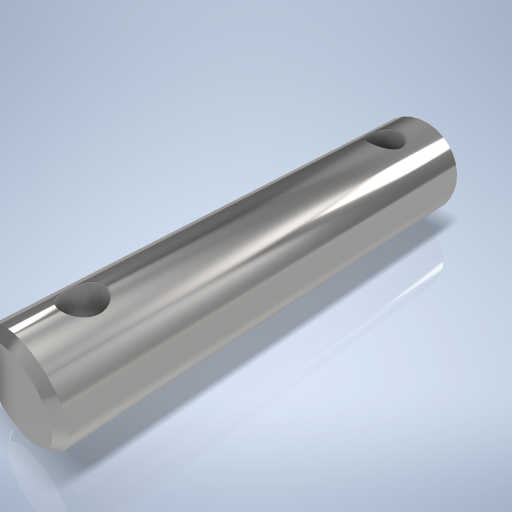
# Autodesk Inventor part: BMS_bolts_left
Saved by Autodesk Inventor 2024.2 (Build 282272000, 272)
## iProperties
Created: 2024-05-14
Part Number: BMS_bolts_left
Material: Edelstahl
Document SubType Name: Modeling
Designer: Fabri
Density: 8 g/cm^3
Appearance: Kordiert 45
Author: Fabri
Autodesk Inventor part; units mm, degrees
ref_plane "YZ Plane" through (0, 0, 0) normal (1, 0, 0) x (0, 1, 0)
ref_plane "XZ Plane" through (0, 0, 0) normal (0, 1, 0) x (-1, 0, 0)
sketch "Skizze1" plane through (0, 0, 0) normal (0, 1, 0) x (-1, 0, 0)
  circle A0 centre (0, 0) radius 3.25
  dimension "d0" = 6.5
  constraints: 1 centre point, 1 coincident
  measures "d0" diameter of A0
extrude "Extrusion1" add sketch "Skizze1" along normal blind 30
chamfer "Fasen1" distance 0.5 angle 45 2 edges at (3.25, 30, 0) (3.25, 0, 0)
ref_plane "Arbeitsebene4" through (0, 0, 3.25) normal (0, 0, 1) x (1, 0, 0)
sketch "Skizze4" plane through (0, 0, 3.25) normal (0, 0, 1) x (1, 0, 0)
  line L0 (-2.75, 30) -> (2.75, 30) projected
  point P0 (0, 0)
  point P1 (0, 4)
  point P2 (0, 26)
  dimension "d25" = 4
  dimension "d26" = 4
  constraints: 2 vertical alignment
  measures "d25" distance of point (0, 4) point (0, 0)
  measures "d26" distance from line of L0 point (0, 26)
hole "Bohrung3" at (0, 4, 3.25) at (0, 26, 3.25) direction (0, 0, -1) diameter 2.5 end through all
